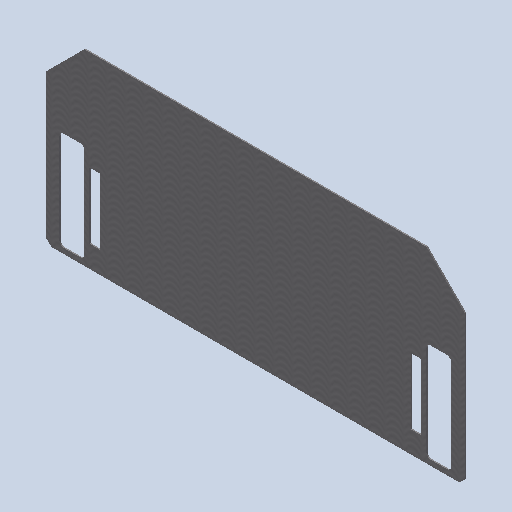
# Autodesk Inventor part: PlanchaBaseInferior
Saved by Autodesk Inventor 2022 (Build 260153000, 153)
## iProperties
Created: 2021-09-22
Part Number: PlanchaBaseInferior
Material: Steel, Mild, Welded
Document SubType Name: Sheet Metal
Designer: Andres
Density: 7.85 g/cm^3
Sheet Metal Rule: Por defecto_mm
Appearance: Weld - Steel Mild
Author: Andres
Autodesk Inventor part; units mm, degrees
ref_plane "YZ Plane" through (0, 0, 0) normal (1, 0, 0) x (0, 1, 0)
ref_plane "XZ Plane" through (0, 0, 0) normal (0, 1, 0) x (-1, 0, 0)
ref_plane "XY Plane" through (0, 0, 0) normal (0, 0, 1) x (1, 0, 0)
sketch "Sketch1" plane through (0, 0, 0) normal (0, 0, 1) x (1, 0, 0)
  line L0 (545.9853, -345.9853) -> (330.9853, -345.9853) construction
  line L1 (545.9853, -370.9853) -> (330.9853, -370.9853) construction
  line L2 (125.9853, -345.9853) -> (750.9853, -345.9853)
  line L3 (750.9853, -345.9853) -> (933.3076, -345.9853)
  line L4 (933.3076, -345.9853) -> (945.9853, -333.3076)
  line L5 (945.9853, -333.3076) -> (945.9853, 16.337)
  line L6 (945.9853, 16.337) -> (853.3076, 109.0147)
  line L7 (853.3076, 109.0147) -> (23.663, 109.0147)
  line L8 (-69.0147, 16.337) -> (23.663, 109.0147)
  line L9 (-69.0147, 16.337) -> (-69.0147, -333.3076)
  line L10 (-69.0147, -333.3076) -> (-56.337, -345.9853)
  line L11 (125.9853, -345.9853) -> (-56.337, -345.9853)
  line L12 (330.9853, -345.9853) -> (330.9853, -370.9853)
  line L13 (545.9853, -345.9853) -> (545.9853, -370.9853)
extrude "Plate1" add sketch "Sketch1" along normal blind 3
sketch "Sketch2" plane through (0, 0, 3) normal (0, 0, 1) x (1, 0, 0)
  line L0 (35.9853, 91.5147) -> (35.9853, -358.4853) projected
  line L1 (60.9853, 91.5147) -> (60.9853, -358.4853) projected
  line L2 (815.9853, 121.5147) -> (815.9853, -358.4853) projected
  line L3 (840.9853, 121.5147) -> (840.9853, -358.4853) projected
  line L4 (-31.5147, -323.1151) -> (-31.5147, -103.1151) projected
  line L5 (18.4853, -103.1151) -> (18.4853, -323.1151) projected
  line L6 (858.0889, -323.1151) -> (858.0889, -103.1151) projected
  line L7 (908.0889, -103.1151) -> (908.0889, -323.1151) projected
  line L8 (-26.5147, -98.1151) -> (13.4853, -98.1151)
  arc A0 (-26.5147, -98.1151) -> (-31.5147, -103.1151) centre (-26.5147, -103.1151) ccw
  arc A1 (18.4853, -103.1151) -> (13.4853, -98.1151) centre (13.4853, -103.1151) ccw
  line L9 (-26.5147, -328.1151) -> (13.4853, -328.1151)
  arc A2 (13.4853, -328.1151) -> (18.4853, -323.1151) centre (13.4853, -323.1151) ccw
  arc A3 (-31.5147, -323.1151) -> (-26.5147, -328.1151) centre (-26.5147, -323.1151) ccw
  arc A4 (903.0889, -328.1151) -> (908.0889, -323.1151) centre (903.0889, -323.1151) ccw
  line L10 (903.0889, -328.1151) -> (863.0889, -328.1151)
  arc A5 (858.0889, -323.1151) -> (863.0889, -328.1151) centre (863.0889, -323.1151) ccw
  arc A6 (908.0889, -103.1151) -> (903.0889, -98.1151) centre (903.0889, -103.1151) ccw
  arc A7 (863.0889, -98.1151) -> (858.0889, -103.1151) centre (863.0889, -103.1151) ccw
  line L11 (903.0889, -98.1151) -> (863.0889, -98.1151)
  line L12 (23.4853, -323.1151) -> (23.4853, -103.1151)
  arc A8 (23.4853, -103.1151) -> (13.4853, -93.1151) centre (13.4853, -103.1151) ccw
  line L13 (13.4853, -93.1151) -> (-26.5147, -93.1151)
  arc A9 (-26.5147, -93.1151) -> (-36.5147, -103.1151) centre (-26.5147, -103.1151) ccw
  line L14 (-36.5147, -103.1151) -> (-36.5147, -323.1151)
  arc A10 (-36.5147, -323.1151) -> (-26.5147, -333.1151) centre (-26.5147, -323.1151) ccw
  line L15 (-26.5147, -333.1151) -> (13.4853, -333.1151)
  arc A11 (13.4853, -333.1151) -> (23.4853, -323.1151) centre (13.4853, -323.1151) ccw
  line L16 (913.0889, -323.1151) -> (913.0889, -103.1151)
  arc A12 (913.0889, -103.1151) -> (903.0889, -93.1151) centre (903.0889, -103.1151) ccw
  line L17 (903.0889, -93.1151) -> (863.0889, -93.1151)
  arc A13 (863.0889, -93.1151) -> (853.0889, -103.1151) centre (863.0889, -103.1151) ccw
  line L18 (853.0889, -103.1151) -> (853.0889, -323.1151)
  arc A14 (853.0889, -323.1151) -> (863.0889, -333.1151) centre (863.0889, -323.1151) ccw
  line L19 (863.0889, -333.1151) -> (903.0889, -333.1151)
  arc A15 (903.0889, -333.1151) -> (913.0889, -323.1151) centre (903.0889, -323.1151) ccw
  line L20 (35.9853, -293.1151) -> (60.9853, -293.1151)
  line L21 (35.9853, -133.1151) -> (60.9853, -133.1151)
  line L22 (840.9853, -133.1151) -> (815.9853, -133.1151)
  line L23 (815.9853, -293.1151) -> (840.9853, -293.1151)
  line L24 (157.9853, 141.0147) -> (157.9853, 99.5147) projected
  line L25 (157.9853, 99.5147) -> (118.9853, 99.5147) projected
  line L26 (118.9853, 99.5147) -> (118.9853, 141.0147) projected
  line L27 (118.9853, 141.0147) -> (157.9853, 141.0147) projected
  point P0 (438.4853, 79.5147)
  dimension "d19" = 5
  dimension "d20" = 5
  dimension "d21" = 40
  dimension "d22" = 40
  dimension "d23" = 40
  dimension "d24" = 40
  constraints: 32 end point, 32 point on circle, 16 centre point, 8 point on line, 5 horizontal, 3 perpendicular, 38 other
  measures "d19" distance between parallel lines of L5 L12
  measures "d20" distance between parallel lines of L7 L16
  measures "d21" distance between parallel lines of L15 L20
  measures "d22" distance between parallel lines of L13 L21
  measures "d23" distance between parallel lines of L17 L22
  measures "d24" distance between parallel lines of L23 L19
extrude "Cut1" cut sketch "Sketch2" against normal through all contours L21 L1 L20 L0 | L22 L3 L23 L2 | L4 A0 L8 A1 L5 A2 L9 A3 | L6 A7 L11 A6 L7 A4 L10 A5 | A11 L15 A10 L14 A9 L13 A8 L12 | A15 L19 A14 L18 A13 L17 A12 L16
equation "\"d6\" = Thickness"
equation "\"d0\" = Thickness"
equation "\"BendRadius\" = Thickness"
equation "\"BendReliefWidth\" = Thickness"
equation "\"BendReliefDepth\" = 0.5 * Thickness"
equation "\"CornerReliefSize\" = 4 * Thickness"
equation "\"MinimumRemnant\" = 2 * Thickness"
equation "\"TransitionRadius\" = BendRadius"
equation "\"JacobiRadiusSize\" = BendRadius"
equation "\"GapSize\" = Thickness"
equation "\"Thickness\" = 3"
body "Solid1"
